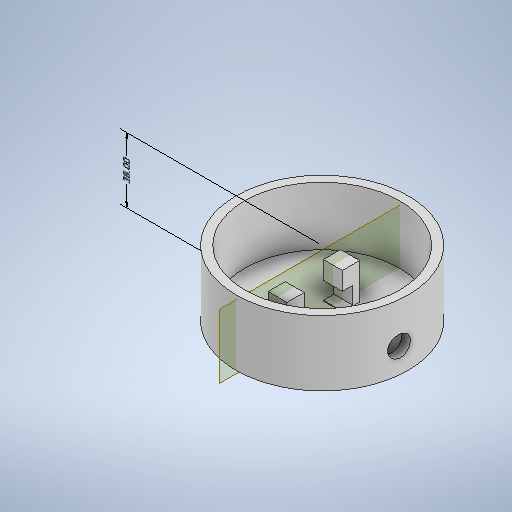
# Autodesk Inventor part: podstawa roobota
Saved by Autodesk Inventor 2025.2 (Build 292293000, 293)
## iProperties
Created: 2025-08-22
Part Number: podstawa roobota
Material: Ogólny
Document SubType Name: Modeling
Designer: IGOR
Density: 1 g/cm^3
Appearance: Domyślna
Author: IGOR
## iProperties of the stored document podstawa roobota_Drukowanie 3D.ipt
Created: 2025-08-25
Part Number: podstawa roobota_Drukowanie 3D
Material: Ogólny
Document SubType Name: Modeling
Designer: IGOR
Density: 1 g/cm^3
Appearance: Domyślna
Author: IGOR
Autodesk Inventor part; units mm, degrees
ref_plane "YZ Plane" through (0, 0, 0) normal (1, 0, 0) x (0, 1, 0)
ref_plane "XZ Plane" through (0, 0, 0) normal (0, 1, 0) x (-1, 0, 0)
ref_plane "XY Plane" through (0, 0, 0) normal (0, 0, 1) x (1, 0, 0)
sketch "Szkic1" plane through (0, 0, 0) normal (0, 1, 0) x (-1, 0, 0)
  circle A0 centre (0, 0) radius 50
  circle A1 centre (0, 0) radius 45
  line L0 (-5.5, 26) -> (5.5, 26)
  line L1 (5.5, 26) -> (5.5, 16)
  line L2 (5.5, 16) -> (-5.5, 16)
  line L3 (-5.5, 16) -> (-5.5, 26)
  line L4 (-5.5, 26) -> (5.5, 16) construction
  line L5 (5.5, 26) -> (-5.5, 16) construction
  line L6 (-5.5, -6.25) -> (5.5, -6.25)
  line L7 (5.5, -6.25) -> (5.5, -16.25)
  line L8 (5.5, -16.25) -> (-5.5, -16.25)
  line L9 (-5.5, -16.25) -> (-5.5, -6.25)
  line L10 (-5.5, -6.25) -> (5.5, -16.25) construction
  line L11 (5.5, -6.25) -> (-5.5, -16.25) construction
  point P0 (0, 21)
  point P1 (0, -11.25)
  point P2 (0, 16)
  dimension "d0" = 100
  dimension "d1" = 90
  dimension "d2" = 11
  dimension "d3" = 10
  dimension "d4" = 11
  dimension "d5" = 10
  dimension "d6" = 6.25
  dimension "d7" = 16
  constraints: 24 end point, 5 midpoint, 4 parallel, 2 centre point, 2 coincident, 2 horizontal, 2 perpendicular
  measures "d0" diameter of A0
  measures "d1" diameter of A1
  measures "d2" distance of L1.end L2.end
  measures "d3" distance of L0.end L1.end
  measures "d4" distance of L7.end L8.end
  measures "d5" distance of L6.end L7.end
  measures "d6" distance from line of point (0, 0) L6
  measures "d7" distance of point (0, 16) point (0, 0)
extrude "Wyciągnięcie proste1" add sketch "Szkic1" along normal blind 25 contours L0 L1 L2 L3 | L6 L7 L8 L9
extrude "Wyciągnięcie proste2" add sketch "Szkic1" along normal blind 38 contours A0
extrude "Wyciągnięcie proste3" add sketch "Szkic1" along normal blind 4 contours A1
sketch "Szkic2" plane through (5.5, 25, 26) normal (1, 0, 0) x (0, 0, -1)
  line L0 (10, -21) -> (10, 0) projected
  line L1 (10, -10.5) -> (4, -10.5)
  line L2 (4, -10.5) -> (4, -20.5)
  line L3 (4, -20.5) -> (10, -20.5)
  line L4 (10, -20.5) -> (10, -10.5)
  line L5 (32.25, -21) -> (32.25, 0) projected
  line L6 (32.25, -10.5) -> (38.25, -10.5)
  line L7 (38.25, -10.5) -> (38.25, -20.5)
  line L8 (38.25, -20.5) -> (32.25, -20.5)
  line L9 (32.25, -20.5) -> (32.25, -10.5)
  point P0 (26, -25)
  point P1 (10, -20.5)
  dimension "d14" = 6
  dimension "d15" = 10
  dimension "d16" = 6
  dimension "d17" = 10
  constraints: 16 end point, 4 parallel, 2 horizontal, 2 midpoint, 2 perpendicular
  measures "d14" distance of L3.end L2.end
  measures "d15" distance of L2.end L1.end
  measures "d16" distance of L7.end L8.end
  measures "d17" distance of L6.end L7.end
extrude "Wyciągnięcie proste4" cut sketch "Szkic2" against normal blind 11
ref_plane "Płaszczyzna konstrukcyjna1" through (0, 25, 16) normal (-1, 0, 0) x (0, 0, 1)
sketch "Szkic3" plane through (0, 25, 16) normal (-1, 0, 0) x (0, 0, 1)
  circle A0 centre (-11.25, -10.5) radius 6
  point P0 (-16, -25)
  dimension "d20" = 12
  constraints: 1 centre point
  measures "d20" diameter of A0
extrude "Wyciągnięcie proste5" cut sketch "Szkic3" against normal through all
sketch "Szkic4" plane through (0, 0, 0) normal (0, -1, 0) x (1, 0, 0)
  point P0 (0, 0)
